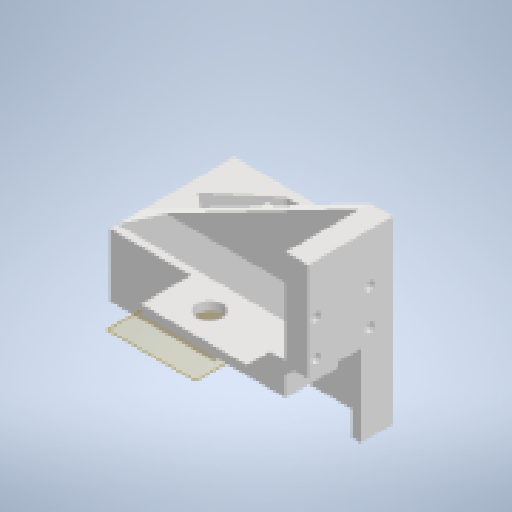
# Autodesk Inventor part: каретка
Saved by Autodesk Inventor 2024.2 (Build 282272000, 272)
## iProperties
Created: 2026-02-13
Part Number: каретка
Material: Типовые
Document SubType Name: Modeling
Designer: Service
Density: 1 g/cm^3
Appearance: По умолчанию
Author: Service
Autodesk Inventor part; units mm, degrees
ref_plane "YZ Plane" through (0, 0, 0) normal (1, 0, 0) x (0, 1, 0)
ref_plane "XZ Plane" through (0, 0, 0) normal (0, 1, 0) x (-1, 0, 0)
ref_plane "РабПлоскость1" through (-7.5749, -280.0826, 223.3085) normal (0, 1, 0) x (-1, 0, 0)
sketch "Эскиз1" plane through (-7.5749, -280.0826, 223.3085) normal (0, 1, 0) x (-1, 0, 0)
  line L0 (14.2093, 4.7851) -> (0, 4.7851)
  line L1 (0, 4.7851) -> (0, -6.2943)
  line L2 (0, -6.2943) -> (14.2093, -6.2943)
  line L3 (14.2093, -6.2943) -> (14.2093, 4.7851)
  line L4 (4.1714, -6.2943) -> (16.1714, -6.2943) projected
  line L5 (0, -6.2943) -> (0, -6.2338) projected
  circle A0 centre (9.1714, -1.5852) radius 2.75 projected
  line L6 (0, -6.2338) -> (-7.9567, -13.9803)
  line L7 (-7.9567, -13.9803) -> (14.2093, -13.9803)
  line L8 (14.2093, -13.9803) -> (14.2093, -6.2943)
  line L9 (-6.416, -12.4803) -> (14.2093, -12.4803)
  line L10 (12.7093, -6.2943) -> (12.7093, -12.4803)
  line L11 (14.2093, 4.7851) -> (18.0834, 4.7851)
  line L12 (18.0834, 4.7851) -> (18.0834, -6.2943)
  line L13 (18.0834, -6.2943) -> (14.2093, -6.2943)
  line L14 (14.2093, -6.2943) -> (14.2093, 4.7851)
  point P0 (-7.5749, -223.3085)
  point P1 (6.5045, -0.9144)
  point P2 (6.5045, -2.256)
  point P3 (0, -6.2338)
  point P4 (12.7093, -6.2943)
  point P5 (14.2093, -6.2943)
  dimension "d2" = 1.5
  dimension "d3" = 1.5
  constraints: 26 end point, 5 perpendicular, 4 parallel, 4 point on line, 3 horizontal, 2 collinear
  measures "d2" distance between parallel lines of L8 L10
  measures "d3" distance between parallel lines of L9 L7
extrude "Выдавливание1" add sketch "Эскиз1" along normal blind 2
extrude "Выдавливание2" add sketch "Эскиз1" against normal blind 12 contours L8 L9 L10 L2 | L8 L7 L6 L9
extrude "Выдавливание3" add sketch "Эскиз1" against normal blind 8 contours L1 L2 L10 L9 L6
sketch "Эскиз2" plane through (-7.5749, -278.0826, 223.3085) normal (0, 1, 0) x (1, 0, 0)
  line L0 (-14.2093, 13.9803) -> (7.9567, 13.9803) projected
  line L1 (-14.2093, 6.2943) -> (-33.1093, 6.2943)
  line L2 (-33.1093, 6.2943) -> (-33.1093, 13.9803)
  line L3 (-33.1093, 13.9803) -> (-14.2093, 13.9803)
  line L4 (-14.2093, 13.9803) -> (-14.2093, 6.2943)
  line L5 (-10.2093, 13.9803) -> (-33.1093, 13.9803)
  line L6 (-33.1093, 13.9803) -> (-33.1093, 33.9803)
  line L7 (-33.1093, 33.9803) -> (-10.2093, 33.9803)
  line L8 (-10.2093, 33.9803) -> (-10.2093, 13.9803)
  circle A0 centre (-19.2093, 22.9803) radius 9
  line L9 (-10.2093, 31.9803) -> (-33.1093, 31.9803)
  line L10 (-33.1093, 22.9803) -> (-22.5164, 31.9803)
  line L11 (-33.1093, 22.9803) -> (-22.5164, 13.9803)
  line L12 (-33.1093, 13.9803) -> (-36.1093, 13.9803)
  line L13 (-36.1093, 13.9803) -> (-36.1093, 33.9803)
  line L14 (-36.1093, 33.9803) -> (-33.1093, 33.9803)
  line L15 (-33.1093, 33.9803) -> (-33.1093, 13.9803)
  point P0 (7.5749, 223.3085)
  point P1 (-12.5164, 13.9803)
  point P2 (-33.1093, 13.9803)
  point P3 (-22.5164, 13.9803)
  dimension "d13" = 20
  dimension "d14" = 18
  dimension "d15" = 2
  dimension "d16" = 18.9
  dimension "d17" = 22.9
  dimension "d18" = 3
  constraints: 30 end point, 7 point on line, 6 parallel, 4 horizontal, 4 tangent, 3 perpendicular, 1 centre point, 1 equal length
  measures "d13" distance of L5.end L6.end
  measures "d14" diameter of A0
  measures "d15" distance between parallel lines of L7 L9
  measures "d16" distance of L2.end L3.end
  measures "d17" distance between parallel lines of L6 L8
  measures "d18" distance between parallel lines of L15 L13
extrude "Выдавливание4" add sketch "Эскиз2" against normal up to surface (14 mm away) contours L4 L1 L2 L3 | L3 L6 L11 | L9 L6 L7 L8 | L12 L13 L14 L6 | L10 L6 L9
sketch "Эскиз3" plane through (-17.7843, -278.0826, 189.3282) normal (0, 0, -1) x (-1, 0, 0)
  line L0 (0, 0) -> (-4.374, 0)
  line L1 (-4.374, 0) -> (-4.374, -14)
  line L2 (-4.374, -14) -> (0, -14)
  line L3 (0, -14) -> (0, 0)
  line L4 (-18.166, -14) -> (-18.166, 0) projected
  line L5 (12.3071, -14) -> (-18.166, -14) projected
  line L6 (-18.166, 0) -> (12.3071, 0) projected
  point P0 (-17.7843, 278.0826)
  constraints: 8 end point, 2 collinear, 2 parallel, 1 horizontal, 1 perpendicular
extrude "Выдавливание5" add sketch "Эскиз3" against normal up to surface (20 mm away) contours L3 L2 L1 L0
sketch "Эскиз4" plane through (-13.4102, -292.0826, 189.3282) normal (1, 0, 0) x (0, 0, -1)
  line L0 (-11, 14) -> (-11, 0) projected
  circle A0 centre (-11, 7) radius 2.1
  point P0 (189.3282, 292.0826)
  dimension "d21" = 4.2
  constraints: 1 centre point, 1 midpoint
  measures "d21" diameter of A0
extrude "Выдавливание6" cut sketch "Эскиз4" against normal up to surface (4.374 mm away)
sketch "Эскиз5" plane through (-7.5749, -278.0826, 223.3085) normal (0, 1, 0) x (1, 0, 0)
  line L0 (7.9567, 13.9803) -> (-5.8353, 13.9803) projected
  line L1 (-10.2979, 13.9803) -> (19.2, 13.9803)
  line L2 (19.2, 13.9803) -> (19.2, 12.4802)
  line L3 (19.2, 12.4802) -> (-10.2979, 12.4802)
  line L4 (-10.2979, 12.4802) -> (-10.2979, 13.9803)
  line L5 (0, -4.7851) -> (0, 6.2338) projected
  point P0 (7.5749, 223.3085)
  point P1 (19.2, 13.2303)
  dimension "d26" = 1.5001
  dimension "d27" = 19.2
  constraints: 8 end point, 2 parallel, 1 horizontal, 1 midpoint, 1 perpendicular, 1 point on line
  measures "d26" distance between parallel lines of L1 L3
  measures "d27" distance from line of L5 point (19.2, 13.23)
extrude "Выдавливание7" add sketch "Эскиз5" against normal up to surface (14 mm away)
sketch "Эскиз6" plane through (-7.5749, -278.0826, 223.3085) normal (0, 1, 0) x (1, 0, 0)
  line L0 (6.4159, 12.4802) -> (19.2, 12.4802) projected
  line L1 (0, 6.2338) -> (6.4159, 12.4802) projected
  line L2 (0, -4.7851) -> (0, 6.2338) projected
  line L3 (0, -4.7851) -> (14.1815, -4.7851)
  line L4 (14.1815, -4.7851) -> (14.1815, -1.2958)
  line L5 (1.5493, -1.2958) -> (1.5493, 6.2338)
  line L6 (1.5493, 6.2338) -> (6.7159, 11.2639)
  line L7 (6.7159, 11.2639) -> (19.2, 11.2639)
  line L8 (19.2, 11.2639) -> (19.2, 12.4802)
  line L9 (19.2, 11.2639) -> (19.2, 6.9814)
  line L10 (19.2, 6.9814) -> (14.1815, 6.9814)
  line L11 (14.1815, 6.9814) -> (14.1815, -1.2958)
  line L12 (1.5493, -1.2958) -> (1.5493, -4.7851)
  line L13 (17.0549, 6.9814) -> (17.0549, 11.2639)
  line L14 (6.7159, 11.2639) -> (6.4159, 12.4802)
  line L15 (17.0549, 11.2639) -> (17.0549, 12.4802)
  point P0 (7.5749, 223.3085)
  constraints: 26 end point, 7 perpendicular, 6 point on line, 1 horizontal, 1 parallel
extrude "Выдавливание8" add sketch "Эскиз6" against normal blind 2
extrude "Выдавливание9" add sketch "Эскиз6" against normal up to surface (14 mm away) contours L0 L8 L7 L15 | L7 L9 L10 L13
sketch "Эскиз7" plane through (-7.5749, -278.0826, 223.3085) normal (0, 1, 0) x (1, 0, 0)
  line L0 (0, 6.2336) -> (12.6363, 6.2336) projected
  line L1 (5.5, 5.0606) -> (17.5, 5.0606) projected
  circle A0 centre (-9.1714, 1.5852) radius 2.75 projected
  line L2 (14.1815, 6.9814) -> (19.2, 6.9814) projected
  line L3 (19.2, 6.9814) -> (19.2, 13.9803) projected
  line L4 (19.2, 13.9803) -> (-5.8353, 13.9803) projected
  line L5 (-5.8353, 33.9803) -> (-5.8353, 13.9803) projected
  line L6 (-5.8353, 33.9803) -> (-36.1093, 33.9803) projected
  line L7 (-36.1093, 33.9803) -> (-36.1093, 13.9803) projected
  line L8 (-36.1093, 13.9803) -> (-33.1093, 13.9803) projected
  line L9 (-33.1093, 13.9803) -> (-33.1093, 6.2943) projected
  line L10 (-33.1093, 6.2943) -> (-18.0834, 6.2943) projected
  line L11 (-18.0834, 6.2943) -> (-18.0834, -4.7851) projected
  line L12 (-18.0834, -4.7851) -> (14.1815, -4.7851) projected
  line L13 (14.1815, -4.7851) -> (14.1815, 6.9814) projected
  line L14 (-10.2093, 13.9803) -> (-22.5164, 13.9803) projected
  line L15 (-22.5164, 13.9803) -> (-33.1093, 22.9803) projected
  line L16 (-33.1093, 22.9803) -> (-22.5164, 31.9803) projected
  line L17 (-22.5164, 31.9803) -> (-10.2093, 31.9803) projected
  line L18 (-10.2093, 31.9803) -> (-10.2093, 13.9803) projected
  line L19 (10.4912, -4.7851) -> (10.4912, 13.9803)
  point P0 (7.5749, 223.3085)
  constraints: 2 end point, 2 point on line, 1 vertical
ref_plane "РабПлоскость2" through (9.6958, -273.9065, 217.0749) normal (0, 1, 0) x (0, 0, 1)
extrude "Выдавливание10" add sketch "Эскиз7" along normal up to surface (4.1761 mm away) contours L19 L4 L3 L2 L13 L1 | L1 L13 L12 L19
sketch "Эскиз8" plane through (2.9163, -273.9065, 209.3282) normal (0, 1, 0) x (1, 0, 0)
  line L0 (8.7088, -6.9989) -> (8.7088, 0) projected
  line L1 (-28.5747, -18.7655) -> (3.6903, -18.7655) projected
  line L2 (8.7088, 0) -> (3.6903, 0)
  line L3 (3.6903, -18.7655) -> (8.7088, -18.7655)
  line L4 (8.7088, -18.7655) -> (8.7088, 0)
  line L5 (8.7088, 0) -> (8.7088, -6.9989) projected
  line L6 (0, 0) -> (8.7088, 0) projected
  line L7 (0, -18.7655) -> (0, 0) projected
  line L8 (3.6903, -18.7655) -> (0, -18.7655) projected
  line L9 (3.6903, -6.9989) -> (3.6903, -18.7655) projected
  line L10 (8.7088, -6.9989) -> (3.6903, -6.9989) projected
  line L11 (3.6903, -6.9989) -> (3.6903, 0)
  point P0 (-2.9163, 209.3282)
  point P1 (3.6903, -18.7655)
  constraints: 8 end point, 1 horizontal, 1 parallel, 1 vertical
extrude "Выдавливание11" add sketch "Эскиз8" along normal blind 22 contours L10 L11 L2 L0 | L4 L3 L9 L10
sketch "Эскиз9" plane through (11.6251, -292.0826, 216.3271) normal (1, 0, 0) x (0, 0, -1)
  circle A0 centre (-3.9716, 15.1761) radius 1.2 projected
  circle A1 centre (-3.3625, 0.1761) radius 1.2 projected
  line L0 (-6.9208, -1.8239) -> (-0.7478, -1.8239) projected
  line L1 (-0.7478, 18.1761) -> (-0.7478, -1.8239) projected
  line L2 (-6.9208, 18.1761) -> (-0.7478, 18.1761) projected
  line L3 (-6.9208, -1.8239) -> (-6.9208, 18.1761) projected
  circle A2 centre (-9.9716, 21.1761) radius 1
  line L4 (-11.7666, 21.1761) -> (6.9989, 21.1761) projected
  circle A3 centre (2.0284, 21.1761) radius 1
  circle A4 centre (-9.9716, 29.1761) radius 1
  circle A5 centre (2.0284, 29.1761) radius 1
  point P0 (216.3271, 292.0826)
  dimension "d38" = 2
  dimension "d39" = 2
  dimension "d40" = 6
  dimension "d41" = 6
  dimension "d42" = 2
  dimension "d43" = 2
  dimension "d45" = 8
  dimension "d46" = 8
  dimension "d47" = 6
  dimension "d48" = 6
  constraints: 4 centre point, 2 point on line
  measures "d38" diameter of A3
  measures "d39" diameter of A2
  measures "d40" horizontal distance of A2.centre A0.centre
  measures "d41" horizontal distance of A3.centre A0.centre
  measures "d42" diameter of A5
  measures "d43" diameter of A4
  measures "d45" distance from line of L4 A5.centre
  measures "d46" distance from line of L4 A4.centre
  measures "d47" horizontal distance of A4.centre A0.centre
  measures "d48" horizontal distance of A0.centre A5.centre
extrude "Выдавливание12" cut sketch "Эскиз9" against normal blind 22 contours L4 A2 | A2 L4 | A3 L4 | L4 A3 | A4 | A5
sketch "Эскиз11" plane through (-13.4102, -292.0826, 209.3282) normal (0, 0, -1) x (-1, 0, 0)
  line L0 (-20.0168, 18.1761) -> (-20.0168, 40.1761) projected
  line L1 (-20.0168, 40.1761) -> (-20.0168, 14)
  line L2 (-20.0168, 14) -> (30.2744, 14)
  line L3 (27.274, 14) -> (12.2481, 14) projected
  line L4 (30.2744, 14) -> (-20.0168, 40.1761)
  point P0 (-13.4102, 292.0826)
  constraints: 6 end point, 1 collinear, 1 perpendicular, 1 vertical
extrude "Выдавливание13" add sketch "Эскиз11" against normal blind 2.25
sketch "Эскиз12" plane through (2.9163, -273.9065, 228.0936) normal (0, 1, 0) x (1, 0, 0)
  line L0 (0, 0) -> (0, 16.5155) projected
  line L1 (3.6903, 11.7666) -> (3.6903, 0) projected
  line L2 (0, 16.5155) -> (3.6903, 16.5155)
  line L3 (3.6903, 16.5155) -> (3.6903, 0)
  line L4 (3.6903, 0) -> (0, 0)
  line L5 (0, 0) -> (0, 16.5155)
  point P0 (-2.9163, 228.0936)
  constraints: 8 end point, 2 parallel, 1 horizontal, 1 perpendicular
extrude "Выдавливание14" add sketch "Эскиз12" along normal blind 1
chamfer "Фаска2" distance 15 angle 45 1 edges at (-15.5973, -278.0826, 209.3282)
chamfer "Фаска3" distance 3.75 angle 45 1 edges at (-18.884, -278.0826, 211.5782)
chamfer "Фаска4" distance 1.75 angle 45 1 edges at (6.6066, -273.9065, 222.2103)
chamfer "Фаска5" distance 5 angle 45 1 edges at (2.9163, -278.0826, 221.7109)
sketch "Эскиз14" plane through (-40.6843, -292.0826, 217.0142) normal (-1, 0, 0) x (0, 0, 1)
  line L0 (-25.6861, 0) -> (-7.6861, 0) projected
  line L1 (-7.6861, 0) -> (0, 0) projected
  line L2 (0, 14) -> (0, 0) projected
  line L3 (-1.6861, 14) -> (0, 14) projected
  line L4 (-7.6861, 14) -> (-1.6861, 14) projected
  line L5 (-7.6861, 14) -> (-7.6861, 0) projected
  point P0 (-217.0142, 292.0826)
extrude "Выдавливание15" add sketch "Эскиз14" along normal up to surface (3 mm away)
sketch "Эскиз15" plane through (-25.6584, -280.0826, 217.0142) normal (0, 0, 1) x (1, 0, 0)
  line L0 (-18.0259, 2) -> (-18.0259, -12) projected
  line L1 (37.2834, -12) -> (12.2481, -12) projected
  line L2 (-18.0259, 0.0767) -> (30.7295, 0.0767)
  line L3 (30.7295, 0.0767) -> (30.7295, -12)
  line L4 (30.7295, -12) -> (-18.0259, -12)
  line L5 (-18.0259, -12) -> (-18.0259, 0.0767)
  point P0 (25.6584, 280.0826)
  point P1 (12.2481, -12)
  constraints: 8 end point, 2 parallel, 2 point on line, 1 horizontal, 1 perpendicular
extrude "Выдавливание16" cut sketch "Эскиз15" against normal blind 2.25
chamfer "Фаска6" distance 2 angle 45 1 edges at (-19.3066, -280.0059, 214.7642)
